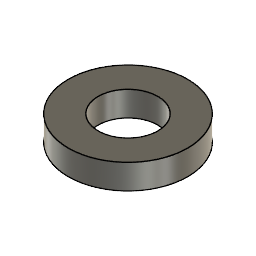
Washer (Autodesk Fusion 360 design; units mm, degrees)
part number: 2026-06-04-11-09-47-763
Autodesk Fusion 360 part; units mm, degrees
sketch "Sketch1" plane through (0, 0, 0) normal (1, 0, 0) x (0, 1, 0)
  line L0 (0, 0) -> (0, 5)
  line L1 (6, 0) -> (12, 0)
  line L2 (12, 0) -> (12, 5)
  line L3 (12, 5) -> (6, 5)
  line L4 (6, 5) -> (6, 0)
  dimension "d7" = 5
  dimension "d8" = 6
  constraint coincident L0.start origin
  constraint vertical L0
  constraint perpendicular L1 L2
  constraint perpendicular L2 L3
  measures "d7" distance of L0.start L0.end
  measures "d8" distance of L1.start L1.end
revolve "Revolve1" add sketch "Sketch1" angle 360 about axis through (0, 0, 0) along (0, 0, 1)
named bodies: "rod bottom cap"
